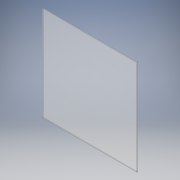
# Autodesk Inventor part: polypropylene_sheet_120x120
Saved by Autodesk Inventor 2019 (Build 230136000, 136)
## iProperties
Created: 2018-10-30
Part Number: polypropylene_sheet_120x120
Material: Polypropylene
Document SubType Name: Modeling
Designer: Gianpietro
Mass: 6.293 g
Surface Area: 143.4 cm^2
Volume: 7 cm^3
Density: 0.899 g/cm^3
Appearance: Smooth - White
Author: Gianpietro
Autodesk Inventor part; units mm, degrees
ref_plane "YZ Plane" through (0, 0, 0) normal (1, 0, 0) x (0, 1, 0)
ref_plane "XZ Plane" through (0, 0, 0) normal (0, 1, 0) x (-1, 0, 0)
ref_plane "XY Plane" through (0, 0, 0) normal (0, 0, 1) x (1, 0, 0)
sketch "Sketch1" plane through (0, 0, 0) normal (0, 0, 1) x (1, 0, 0)
  line L0 (-60, -60) -> (60, -60)
  line L1 (60, -60) -> (60, 60)
  line L2 (60, 60) -> (-60, 60)
  line L3 (-60, 60) -> (-60, -60)
  line L4 (-60, -60) -> (60, 60) construction
  line L5 (60, -60) -> (-60, 60) construction
  point P0 (0, 0)
  dimension "d0" = 120
  dimension "d1" = 120
  constraints: 12 end point, 2 midpoint, 2 parallel, 1 horizontal, 1 perpendicular
  measures "d0" distance of L2.end L1.end
  measures "d1" distance of L1.end L0.end
extrude "Extrusion1" add sketch "Sketch1" along normal blind 1
body "Solid1"
